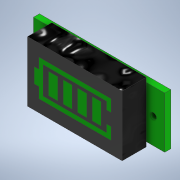
# Autodesk Inventor part: Измеритель заряда
Saved by Autodesk Inventor 2022 (Build 260153000, 153)
## iProperties
Created: 2022-06-08
Part Number: Измеритель заряда
Material: Типовые
Document SubType Name: Modeling
Designer: Admin
Density: 1 g/cm^3
Appearance: По умолчанию
Author: Admin
Autodesk Inventor part; units mm, degrees
ref_plane "YZ Plane" through (0, 0, 0) normal (1, 0, 0) x (0, 1, 0)
ref_plane "XZ Plane" through (0, 0, 0) normal (0, 1, 0) x (-1, 0, 0)
ref_plane "XY Plane" through (0, 0, 0) normal (0, 0, 1) x (1, 0, 0)
sketch "Эскиз1" plane through (0, 0, 0) normal (0, 0, 1) x (1, 0, 0)
  line L0 (15.65, 10) -> (-15.65, 10)
  line L1 (-15.65, 10) -> (-15.65, -10)
  line L2 (-15.65, -10) -> (15.65, -10)
  line L3 (15.65, -10) -> (15.65, 10)
  line L4 (15.65, 10) -> (-15.65, -10) construction
  line L5 (-15.65, 10) -> (15.65, -10) construction
  line L6 (-21.75, 8.5) -> (21.75, 8.5)
  line L7 (21.75, 8.5) -> (21.75, -8.5)
  line L8 (21.75, -8.5) -> (-21.75, -8.5)
  line L9 (-21.75, -8.5) -> (-21.75, 8.5)
  line L10 (-21.75, 8.5) -> (21.75, -8.5) construction
  line L11 (21.75, 8.5) -> (-21.75, -8.5) construction
  circle A0 centre (-18, 0) radius 1
  circle A1 centre (18, 0) radius 1
  point P0 (0, 0)
  point P1 (0, 0)
  dimension "d0" = 31.3
  dimension "d1" = 20
  dimension "d2" = 43.5
  dimension "d3" = 17
  dimension "d4" = 2
  dimension "d5" = 2
  dimension "d6" = 36
  dimension "d7" = 18
  constraints: 24 end point, 5 midpoint, 4 parallel, 2 centre point, 2 horizontal, 2 horizontal alignment, 2 perpendicular
  measures "d0" distance of L2.end L1.end
  measures "d1" distance of L1.end L0.end
  measures "d2" distance of L7.end L8.end
  measures "d3" distance of L6.end L7.end
  measures "d4" diameter of A0
  measures "d5" diameter of A1
  measures "d6" distance of A0.centre A1.centre
  measures "d7" distance of point (0, 0) A1.centre
extrude "Выдавливание1" add sketch "Эскиз1" along normal blind 8 contours L3 L6 L1 L0 | L3 L8 L1 L6 | L3 L2 L1 L8
extrude "Выдавливание2" add sketch "Эскиз1" against normal blind 2 contours L6 L7 L8 L3 | L3 L8 L1 L6 | L1 L8 L9 L6 | A0 | A1
extrude "Выдавливание3" cut sketch "Эскиз1" against normal through all contours A0 | A1
sketch "Эскиз2" plane through (0, 0, 8) normal (0, 0, 1) x (1, 0, 0)
  line L0 (12, -6) -> (-12, -6)
  line L1 (-12, -6) -> (-12, -2.5)
  line L2 (-12, -2.5) -> (-13.5, -2.5)
  line L3 (-13.5, -2.5) -> (-13.5, 2.5)
  line L4 (-13.5, 2.5) -> (-12, 2.5)
  line L5 (-12, 2.5) -> (-12, 6)
  line L6 (-12, 6) -> (12, 6)
  line L7 (12, 6) -> (12, 2)
  line L8 (12, 2) -> (10.5, 2)
  line L9 (10.5, 4.5) -> (-10.5, 4.5)
  line L10 (-10.5, 4.5) -> (-10.5, -4.5)
  line L11 (-10.5, -4.5) -> (10.5, -4.5)
  line L12 (10.5, -4.5) -> (10.5, -2)
  line L13 (10.5, -2) -> (12, -2)
  line L14 (12, -2) -> (12, -6)
  line L15 (10.5, 4.5) -> (10.5, 2)
  line L16 (8.7, 3.5) -> (5.7, 3.5)
  line L17 (5.7, 3.5) -> (5.7, -3.5)
  line L18 (5.7, -3.5) -> (8.7, -3.5)
  line L19 (8.7, -3.5) -> (8.7, 3.5)
  line L20 (8.7, 3.5) -> (5.7, -3.5) construction
  line L21 (5.7, 3.5) -> (8.7, -3.5) construction
  line L22 (3.9, 3.5) -> (0.9, 3.5)
  line L23 (0.9, 3.5) -> (0.9, -3.5)
  line L24 (0.9, -3.5) -> (3.9, -3.5)
  line L25 (3.9, -3.5) -> (3.9, 3.5)
  line L26 (3.9, 3.5) -> (0.9, -3.5) construction
  line L27 (0.9, 3.5) -> (3.9, -3.5) construction
  line L28 (-0.9, 3.5) -> (-3.9, 3.5)
  line L29 (-3.9, 3.5) -> (-3.9, -3.5)
  line L30 (-3.9, -3.5) -> (-0.9, -3.5)
  line L31 (-0.9, -3.5) -> (-0.9, 3.5)
  line L32 (-0.9, 3.5) -> (-3.9, -3.5) construction
  line L33 (-3.9, 3.5) -> (-0.9, -3.5) construction
  line L34 (-5.7, 3.5) -> (-8.7, 3.5)
  line L35 (-8.7, 3.5) -> (-8.7, -3.5)
  line L36 (-8.7, -3.5) -> (-5.7, -3.5)
  line L37 (-5.7, -3.5) -> (-5.7, 3.5)
  line L38 (-5.7, 3.5) -> (-8.7, -3.5) construction
  line L39 (-8.7, 3.5) -> (-5.7, -3.5) construction
  point P0 (0, 0)
  point P1 (-13.5, 0)
  point P2 (-10.5, 0)
  point P3 (7.2, 0)
  point P4 (2.4, 0)
  point P5 (-2.4, 0)
  point P6 (-7.2, 0)
  point P7 (-7.2, 0)
  point P8 (-2.4, 0)
  point P9 (-2.4, 0)
  point P10 (2.4, 0)
  point P11 (2.4, 0)
  point P12 (7.2, 0)
  point P13 (7.2, 0)
  point P14 (0, -6)
  dimension "d14" = 1.5
  dimension "d15" = 1.5
  dimension "d16" = 1.5
  dimension "d17" = 1.5
  dimension "d18" = 3
  dimension "d19" = 5
  dimension "d20" = 12
  dimension "d21" = 4
  dimension "d22" = 3
  dimension "d23" = 7
  dimension "d24" = 1.8
  dimension "d25" = 1.8
  dimension "d26" = 1.8
  dimension "d28" = 1.8
  dimension "d29" = 1.8
  constraints: 80 end point, 18 midpoint, 14 perpendicular, 9 equal length, 8 parallel, 6 horizontal alignment, 5 horizontal, 5 point on line, 3 vertical, 1 vertical alignment
  measures "d14" distance between parallel lines of L0 L11
  measures "d15" distance between parallel lines of L14 L12
  measures "d16" distance of L7.end L8.end
  measures "d17" distance between parallel lines of L1 L10
  measures "d18" distance between parallel lines of L10 L3
  measures "d19" distance of L2.end L3.end
  measures "d20" distance of L5.end L0.end
  measures "d21" distance between parallel lines of L8 L13
  measures "d22" distance of L35.end L36.end
  measures "d23" distance of L36.end L34.start
  measures "d24" distance between parallel lines of L10 L35
  measures "d25" distance between parallel lines of L12 L19
  measures "d26" distance between parallel lines of L17 L25
  measures "d28" distance between parallel lines of L23 L31
  measures "d29" distance between parallel lines of L37 L29
extrude "Выдавливание4" cut sketch "Эскиз2" against normal blind 1
extrude "Выдавливание5" add sketch "Эскиз2" against normal blind 1 separate body
